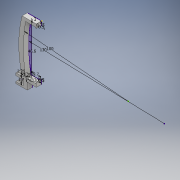
# Autodesk Inventor part: RightClip
Saved by Autodesk Inventor 2019 (Build 230136000, 136)
## iProperties
Created: 2017-12-02
Part Number: RightClip
Material: Generic
Document SubType Name: Modeling
Designer: Max
Density: 1 g/cm^3
Appearance: Default
Author: Max
Autodesk Inventor part; units mm, degrees
ref_plane "YZ Plane" through (0, 0, 0) normal (1, 0, 0) x (0, 1, 0)
ref_plane "XZ Plane" through (0, 0, 0) normal (0, 1, 0) x (-1, 0, 0)
ref_plane "XY Plane" through (0, 0, 0) normal (0, 0, 1) x (1, 0, 0)
sketch "Sketch1" plane through (0, 0, 0) normal (0, 1, 0) x (-1, 0, 0)
  line L0 (10.2, -3) -> (10.2, -49.6)
  line L1 (10.2, -49.6) -> (0.5, -49.6)
  line L2 (0.5, -49.6) -> (0.5, -48.85)
  line L3 (0.5, -48.85) -> (0, -48.85)
  line L4 (0, -48.85) -> (0, -49.6)
  line L5 (0.5, -3) -> (0.5, -3.75)
  line L6 (0.5, -3.75) -> (0, -3.75)
  line L7 (0, -3.75) -> (0, -3)
  line L8 (0, -3) -> (0, 0)
  line L9 (0, 0) -> (13.5647, 0)
  line L10 (13.2, -52.6) -> (12.7, -52.6)
  line L11 (0, -52.6) -> (0, -49.6)
  line L12 (10.2, -3) -> (0.5, -3)
  line L13 (8.7, -59.3) -> (19.7, -59.3)
  line L14 (19.7, -59.3) -> (19.7, -57.6)
  line L15 (19.7, -57.6) -> (12.7, -57.6)
  line L16 (12.7, -57.6) -> (12.7, -52.6)
  line L17 (12.7, -52.6) -> (13.2, -52.6)
  line L18 (19.7, -52.6) -> (19.7, -50.35)
  line L19 (19.7, -50.35) -> (13.5647, -50.35)
  line L20 (8.7, -59.3) -> (8.7, -52.6)
  arc A0 (10.2, -49.6) -> (10.2, -3) centre (-117.6949, -26.3) ccw
  line L21 (12.7, -52.6) -> (12.7, -52.6)
  line L22 (13.2, -52.6) -> (19.7, -52.6)
  line L23 (13.2, -52.6) -> (13.2, -52.6)
  line L24 (8.7, -52.6) -> (0, -52.6)
  arc A1 (13.5647, -50.35) -> (13.5647, 0) centre (-83.2145, -25.175) ccw
  point P0 (0, 0)
  dimension "d1" = 9.7
  dimension "d2" = 0.75
  dimension "d3" = 0.5
  dimension "d6" = 0.5
  dimension "d10" = 46.6
  dimension "d13" = 0.75
  dimension "d14" = 3
  dimension "d15" = 3
  dimension "d16" = 5
  dimension "d19" = 7
  dimension "d25" = 130
  dimension "d30" = 2.25
  dimension "d31" = 2.25
  dimension "d32" = 1.7
  dimension "d33" = 4
  dimension "d34" = 100
  dimension "d35" = 12.7
  constraints: 50 end point, 24 perpendicular, 6 point on line, 4 point on circle, 2 centre point, 2 horizontal, 1 coincident, 1 parallel
  measures "d1" distance of L0.end L1.end
  measures "d2" distance of L1.end L2.end
  measures "d3" distance of L2.end L3.end
  measures "d6" distance of L5.end L6.end
  measures "d10" distance of L0.start L0.end
  measures "d13" distance between parallel lines of L6 L12
  measures "d14" distance between parallel lines of L9 L12
  measures "d15" distance between parallel lines of L10 L1
  measures "d16" distance of L15.end L17.start
  measures "d19" distance of L17.start L18.start
  measures "d25" radius of A0
  measures "d30" distance from line of L10 L19.end
  measures "d31" distance of L18.start L18.end
  measures "d32" distance of L13.end L14.end
  measures "d33" distance between parallel lines of L20 L16
  measures "d34" radius of A1
  measures "d35" distance between parallel lines of L16 L11
extrude "Extrusion2" add sketch "Sketch1" against normal blind 5 contours L12 L5 L6 L7 L8 L9 A1 L19 L18 L22 L10 L16 L15 L14 L13 L20 L24 L11 L4 L3 L2 L1 A0
body "Solid1"
